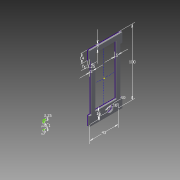
# Autodesk Inventor part: body-side2
Saved by Autodesk Inventor 2013 (Build 170138000, 138)
## iProperties
Created: 2012-09-08
Part Number: body-side2
Material: Generic
Document SubType Name: Modeling
Designer: frankenteddy
Density: 1 g/cm^3
Author: frankenteddy
Autodesk Inventor part; units mm, degrees
ref_plane "YZ Plane" through (0, 0, 0) normal (1, 0, 0) x (0, 1, 0)
ref_plane "XZ Plane" through (0, 0, 0) normal (0, 1, 0) x (-1, 0, 0)
ref_plane "XY Plane" through (0, 0, 0) normal (0, 0, 1) x (1, 0, 0)
sketch "Sketch1" plane through (0, 0, 0) normal (1, 0, 0) x (0, 1, 0)
  line L0 (-92.7646, -8.503) -> (-89.7646, -8.503)
  line L1 (-89.7646, -8.503) -> (-89.7646, -11.753)
  line L2 (-89.7646, -11.753) -> (-92.7646, -11.753)
  line L3 (-92.7646, -11.753) -> (-92.7646, -8.503)
  line L4 (-92.7646, -21.6527) -> (-89.7646, -21.6527)
  line L5 (-89.7646, -21.6527) -> (-89.7646, -21.7527)
  line L6 (-89.7646, -21.7527) -> (-92.7646, -21.7527)
  line L7 (-92.7646, -21.7527) -> (-92.7646, -21.6527)
  line L8 (-21.5, 50) -> (21.5, 50)
  line L9 (21.5, 50) -> (21.5, -50)
  line L10 (21.5, -50) -> (-21.5, -50)
  line L11 (-21.5, -50) -> (-21.5, 50)
  line L12 (0, 50) -> (0, -50) construction
  line L13 (-21.5, 0) -> (21.5, 0) construction
  line L14 (-16.5, 43) -> (16.5, 43)
  line L15 (16.5, 43) -> (16.5, -34)
  line L16 (16.5, -34) -> (-16.5, -34)
  line L17 (-16.5, -34) -> (-16.5, 43)
  circle A0 centre (6.5, -42) radius 5
  line L18 (-21.5, 50) -> (-24.75, 50)
  line L19 (-24.75, 50) -> (-24.75, 36)
  line L20 (-24.75, 36) -> (-21.5, 36)
  line L21 (-21.5, 36) -> (-21.5, 50)
  line L22 (21.5, 50) -> (24.75, 50)
  line L23 (24.75, 50) -> (24.75, 36)
  line L24 (24.75, 36) -> (21.5, 36)
  line L25 (21.5, 36) -> (21.5, 50)
  line L26 (-21.5, -50) -> (-24.75, -50)
  line L27 (-24.75, -50) -> (-24.75, -36)
  line L28 (-24.75, -36) -> (-21.5, -36)
  line L29 (-21.5, -36) -> (-21.5, -50)
  line L30 (21.5, -36) -> (21.5, -50)
  line L31 (24.75, -50) -> (24.75, -36)
  line L32 (24.75, -36) -> (21.5, -36)
  line L33 (21.5, -50) -> (24.75, -50)
  point P0 (0, 0)
  dimension "d0" = 3
  dimension "mat" = 3.25
  dimension "d2" = 3
  dimension "kerf" = 0.1
  dimension "d4" = 43
  dimension "d5" = 100
  dimension "d9" = 7
  dimension "d10" = 16
  dimension "d11" = 5
  dimension "d12" = 5
  dimension "d13" = 10
  dimension "d15" = 3
  dimension "d16" = 3.25
  dimension "d17" = 14
  dimension "d24" = 10
  constraints: 68 end point, 10 parallel, 9 symmetric about line, 6 midpoint, 5 horizontal, 5 perpendicular, 1 centre point
  measures "d0" distance of L1.end L2.end
  measures "mat" distance of L0.end L1.end
  measures "d2" distance of L5.end L6.end
  measures "kerf" distance of L4.end L5.end
  measures "d4" distance of L9.end L10.end
  measures "d5" distance of L8.end L9.end
  measures "d9" distance between parallel lines of L14 L8
  measures "d10" distance between parallel lines of L16 L10
  measures "d11" distance between parallel lines of L17 L11
  measures "d12" distance between parallel lines of L9 L15
  measures "d13" diameter of A0
  measures "d15" distance edge to line of A0 L10
  measures "d16" distance of L20.end L19.end
  measures "d17" distance of L19.end L18.end
  measures "d24" distance edge to line of A0 L9
extrude "Extrusion1" [suppressed]
extrude "Extrusion2" add sketch "Sketch1" along normal blind 3.25 contours L11 L20 L19 L18 | L22 L23 L24 L9 | L11 L26 L27 L28 | L32 L31 L33 L9
extrude "Extrusion3" add sketch "Sketch1" along normal blind 3.25 contours L8 L9 L10 L11
equation "\"d16\" = mat"
equation "\"d18\" = mat"
equation "\"d20\" = mat"
equation "\"d22\" = mat"
body "Solid1"
